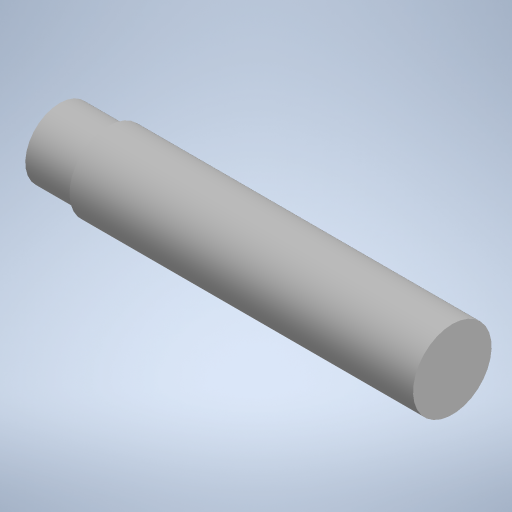
# Autodesk Inventor part: LJ12
Saved by Autodesk Inventor 2023 (Build 270158000, 158)
## iProperties
Created: 2022-05-30
Part Number: LJ12
Material: Generic
Document SubType Name: Modeling
Designer: plebbb
Density: 1 g/cm^3
Appearance: Default
Author: plebbb
Autodesk Inventor part; units mm, degrees
ref_plane "YZ Plane" through (0, 0, 0) normal (1, 0, 0) x (0, 1, 0)
ref_plane "XZ Plane" through (0, 0, 0) normal (0, 1, 0) x (-1, 0, 0)
ref_plane "XY Plane" through (0, 0, 0) normal (0, 0, 1) x (1, 0, 0)
sketch "Sketch1" plane through (0, 0, 0) normal (0, 0, 1) x (1, 0, 0)
  line L0 (0, 0) -> (0, 5.25)
  line L1 (0, 5.25) -> (7.5, 5.25)
  line L2 (7.5, 5.25) -> (7.5, 6)
  line L3 (7.5, 6) -> (60, 6)
  line L4 (60, 6) -> (60, 0)
  line L5 (60, 0) -> (0, 0)
  point P0 (60, 3)
  point P1 (0, 2.625)
  dimension "d0" = 6
  dimension "d1" = 5.25
  dimension "d2" = 7.5
  dimension "d3" = 60
  constraints: 12 end point, 3 perpendicular, 2 midpoint, 2 parallel, 1 vertical
  measures "d0" distance of L3.end L4.end
  measures "d1" distance of L0.start L0.end
  measures "d2" distance of L0.end L1.end
  measures "d3" horizontal distance of point (60, 3) point (0, 2.625)
revolve "Revolution1" add sketch "Sketch1" angle 360 about axis through (60, 0, 0) along (-1, 0, 0)
body "Solid1"
